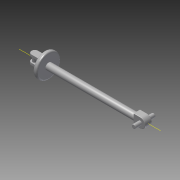
# Autodesk Inventor part: Follower
Saved by Autodesk Inventor 2015 (Build 190141000, 141)
## iProperties
Created: 2008-06-13
Part Number: Follower
Document SubType Name: Modeling
Designer: tangg
Density: 7.85 g/cm^3
Mass: 2.02034 g
Surface Area: 17.8273 cm^2
Volume: 2.02034 cm^3
Stock Number: Follower
Material: Alloy Steel
Appearance: Steel
Author: tangg
Autodesk Inventor part; units mm, degrees
ref_plane "XZ Plane" through (0, 0, 0) normal (0, 1, 0) x (-1, 0, 0)
ref_plane "XY Plane" through (0, 0, 0) normal (0, 0, 1) x (1, 0, 0)
sketch "Sketch1" plane through (0, 0, 0) normal (0, 0, 1) x (1, 0, 0)
  line L0 (0, 3.75) -> (-82.55, 3.75)
  line L1 (-82.55, 3.75) -> (-82.55, -3.75)
  line L2 (-82.55, -3.75) -> (0, -3.75)
  line L3 (0, -3.75) -> (0, 3.75)
  circle A0 centre (0, 0) radius 3.75
  dimension "d0" = 7.5
  dimension "d1" = 82.55
  constraints: 8 end point, 3 perpendicular, 1 coincident, 1 midpoint, 1 vertical, 1 vertical alignment, 2 other
  measures "d0" distance of L2.end L0.start
  measures "d1" distance of L1.end L2.end
extrude "Extrusion1" add sketch "Sketch1" along normal mid plane 5.08
ref_plane "Work Plane4" through (-5.08, 0, 0) normal (1, 0, 0) x (0, 1, 0)
sketch "Sketch16" plane through (-5.08, 0, 0) normal (1, 0, 0) x (0, 1, 0)
  circle A0 centre (0, 0) radius 2.54
  line L0 (3.75, 2.54) -> (3.75, -2.54) projected
  line L1 (3.75, -2.54) -> (-3.75, -2.54) projected
  line L2 (-3.75, -2.54) -> (-3.75, 2.54) projected
  line L3 (-3.75, 2.54) -> (3.75, 2.54) projected
  dimension "d28" = 5.08
  constraints: 1 centre point, 1 coincident
  measures "d28" diameter of A0
extrude "Extrusion11" cut sketch "Sketch16" against normal blind 69.85 contours A0 L3 L0 L1 | A0 L1 L2 L3
sketch "Sketch2" plane through (0, 0, 0) normal (0, 0, 1) x (1, 0, 0)
  circle A0 centre (0, 0) radius 1.5
  dimension "d32" = 3
  constraints: 1 centre point, 1 coincident
  measures "d32" diameter of A0
extrude "Extrusion2" add sketch "Sketch2" along normal mid plane 15.24
sketch "Sketch11" plane through (0, 0, 0) normal (0, 1, 0) x (-1, 0, 0)
  circle A0 centre (82.55, 0) radius 2.54
  line L0 (82.55, -2.54) -> (82.55, 2.54) projected
  line L1 (82.55, -2.54) -> (82.55, 2.54) projected
  point P0 (0, 0)
  constraints: 1 centre point, 1 coincident, 1 midpoint
extrude "Extrusion7" add sketch "Sketch11" along normal mid plane 7.5
sketch "Sketch12" plane through (0, 0, 0) normal (0, 1, 0) x (-1, 0, 0)
  circle A0 centre (82.55, 0) radius 4.7625
  line L0 (5.08, -2.54) -> (0, -2.54) projected
  arc A1 (82.55, -2.54) -> (82.55, 2.54) centre (82.55, 0) ccw projected
  arc A2 (82.55, -2.54) -> (82.55, 2.54) centre (82.55, 0) ccw projected
  point P0 (0, 0)
  constraints: 1 centre point, 1 coincident
extrude "Extrusion8" cut sketch "Sketch12" against normal mid plane 3.81
sketch "Sketch15" plane through (0, 0, 0) normal (0, 1, 0) x (-1, 0, 0)
  circle A0 centre (82.55, 0) radius 1.5875
  arc A1 (82.55, -2.54) -> (82.55, 2.54) centre (82.55, 0) ccw projected
  point P0 (0, 0)
  point P1 (80.645, -1.6801)
  point P2 (80.645, 1.6801)
  constraints: 1 centre point, 1 coincident
extrude "Extrusion10" add sketch "Sketch15" along normal mid plane 5.08
fillet "Fillet2" radius 0.3175 14 edges at (-2.54, -3.75, 2.54) (-78.74, -3.75, 2.54) (3.75, 0, 2.54) (-2.54, 3.75, 2.54) (-78.74, 3.75, 2.54) (-2.54, 3.75, -2.54) (-78.74, 3.75, -2.54) (-2.54, -3.75, -2.54) (-78.74, -3.75, -2.54) (3.75, 0, -2.54) (-85.09, -3.75, 0) (-85.09, 3.75, 0) (-1.5, 0, 7.62) (-1.5, 0, -7.62)
sketch "Sketch17" plane through (-74.93, 0, 0) normal (1, 0, 0) x (0, 0, -1)
  circle A0 centre (0, 0) radius 9
  dimension "d36" = 18
  constraints: 1 centre point, 1 coincident
  measures "d36" diameter of A0
extrude "Extrusion12" add sketch "Sketch17" along normal blind 3
fillet "Fillet4" radius 1 10 edges at (-74.93, 3.75, 0) (-74.93, 3.657, -2.447) (-74.93, 0, -2.54) (-74.93, -3.657, -2.447) (-74.93, -3.75, 0) (-74.93, -3.657, 2.447) (-74.93, 0, 2.54) (-74.93, 3.657, 2.447) (-74.93, 0, 9) (-71.93, 0, 9)
body "Solid1"
